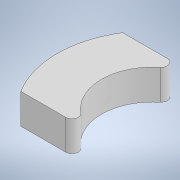
# Autodesk Inventor part: Crank Insert
Saved by Autodesk Inventor 2022.2 (Build 262287000, 287)
## iProperties
Created: 2022-08-14
Part Number: Crank Insert
Material: Generic
Document SubType Name: Modeling
Designer: Ilewicz
Density: 1 g/cm^3
Appearance: Default
Author: Ilewicz
Autodesk Inventor part; units mm, degrees
ref_plane "YZ Plane" through (0, 0, 0) normal (1, 0, 0) x (0, 1, 0)
ref_plane "XZ Plane" through (0, 0, 0) normal (0, 1, 0) x (-1, 0, 0)
ref_plane "XY Plane" through (0, 0, 0) normal (0, 0, 1) x (1, 0, 0)
derived "Crank.ipt"
sketch "Sketch1" plane through (0, 0, 0) normal (0, 1, 0) x (-1, 0, 0)
  arc A0 (0, -8) -> (0, 8) centre (0, 0) ccw
  line L0 (0, 8) -> (12.6886, 8)
  line L1 (0, -8) -> (12.6886, -8)
  arc A1 (12.6886, -8) -> (12.6886, 8) centre (0, 0) ccw
  dimension "d0" = 8
  dimension "d2" = 15
  constraints: 4 end point, 4 point on circle, 2 centre point, 2 coincident, 2 horizontal, 1 tangent
  measures "d0" radius of A0
  measures "d2" radius of A1
extrude "Extrusion1" add sketch "Sketch1" along normal blind 4.75
fillet "Fillet1" radius 1 2 edges at (0, 2.375, 8) (0, 2.375, -8)
equation "\"d2\" = r_crank"
equation "\"r_crank\" = 15"
body "Solid1"
